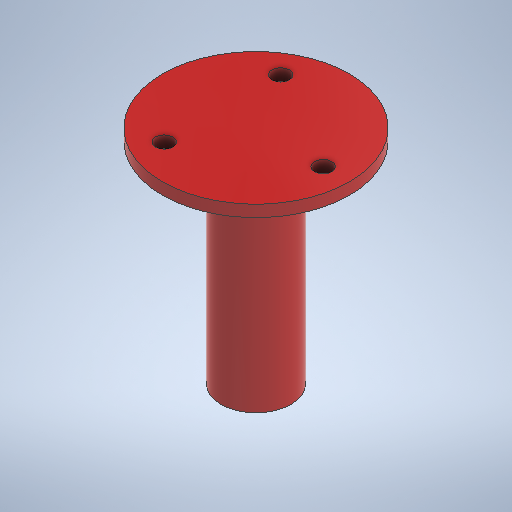
# Autodesk Inventor part: Motorbefestigung
Saved by Autodesk Inventor 2025.1 (Build 291241000, 241)
## iProperties
Created: 2024-12-04
Part Number: Motorbefestigung
Material: Generisch
Document SubType Name: Modeling
Designer: Julian
Density: 1 g/cm^3
Appearance: Vorgabe
Author: Julian
Autodesk Inventor part; units mm, degrees
ref_plane "YZ Plane" through (0, 0, 0) normal (1, 0, 0) x (0, 1, 0)
ref_plane "XZ Plane" through (0, 0, 0) normal (0, 1, 0) x (-1, 0, 0)
ref_plane "XY Plane" through (0, 0, 0) normal (0, 0, 1) x (1, 0, 0)
sketch "Skizze1" plane through (0, 0, 0) normal (0, 0, 1) x (1, 0, 0)
  circle A0 centre (0, 0) radius 16
  dimension "d0" = 32
  constraints: 1 centre point, 1 coincident
  measures "d0" diameter of A0
extrude "Befestigungsfläche" add sketch "Skizze1" along normal blind 2
sketch "Skizze2" plane through (0, 0, 0) normal (0, 0, -1) x (-1, 0, 0)
  circle A0 centre (0, 0) radius 7
  dimension "d4" = 14
  constraints: 1 centre point, 1 coincident
  measures "d4" diameter of A0
extrude "Mittelfläche" add sketch "Skizze2" along normal blind 2
sketch "Skizze3" plane through (0, 0, -2) normal (0, 0, -1) x (-1, 0, 0)
  circle A0 centre (0, 0) radius 6
  dimension "d7" = 12
  constraints: 1 centre point, 1 coincident
  measures "d7" diameter of A0
extrude "Hauptkörper" add sketch "Skizze3" along normal blind 34
sketch "Skizze4" plane through (0, 0, -36) normal (0, 0, -1) x (-1, 0, 0)
  arc A0 (-0.1762, -1.9922) -> (-1.9922, -0.1762) centre (0, 0) ccw
  line L0 (-1.9922, -0.1762) -> (-0.1762, -1.9922)
  dimension "d10" = 4
  constraints: 2 end point, 2 point on circle, 1 centre point, 1 coincident
  measures "d10" diameter of A0
extrude "Motorschaft (negativ)" cut sketch "Skizze4" against normal blind 10
sketch "Skizze6" plane through (0, 0, 2) normal (0, 0, 1) x (1, 0, 0)
  circle A0 centre (0, 0) radius 7
  line L0 (0, 0) -> (11.5, 0) construction
  line L1 (0, 0) -> (11.5, 0) construction
  circle A1 centre (11.5, 0) radius 1.5
  circle A2 centre (-5.75, 9.9593) radius 1.5
  circle A3 centre (-5.75, -9.9593) radius 1.5
  line L2 (0, 0) -> (11.5, 0)
  line L3 (0, 0) -> (-5.75, -9.9593)
  line L4 (0, 0) -> (11.5, 0) construction
  line L5 (0, 0) -> (-5.75, 9.9593)
  line L6 (0, 0) -> (11.5, 0) construction
  dimension "d14" = 14
  dimension "d21" = 3
  dimension "d22" = 3
  dimension "d23" = 3
  dimension "d26" = 11.5
  dimension "d27" = 11.5
  dimension "d28" = 120
  dimension "d29" = 11.5
  dimension "d30" = 120
  constraints: 15 end point, 4 centre point, 4 horizontal, 3 coincident, 2 equal length
  measures "d14" diameter of A0
  measures "d21" diameter of A1
  measures "d22" diameter of A2
  measures "d23" diameter of A3
  measures "d26" distance of L0.start L0.end
  measures "d27" distance of L0.start L3.end
  measures "d28" angle of L3 L4
  measures "d29" distance of L0.start L5.end
  measures "d30" angle of L6 L5
extrude "Löcher" cut sketch "Skizze6" against normal blind 2 contours A3 | A2 | A1
